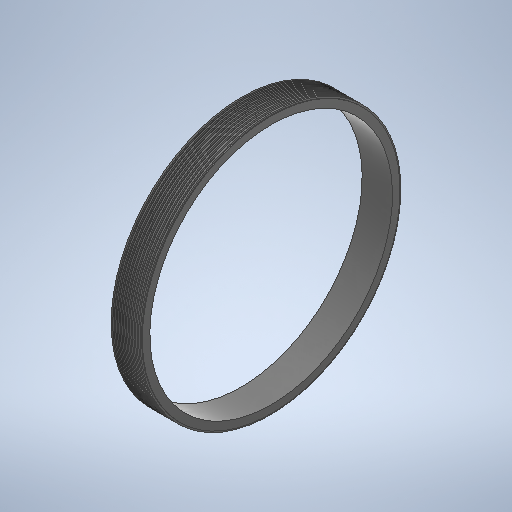
# Autodesk Inventor part: TPU Tire
Saved by Autodesk Inventor 2025.2 (Build 292293000, 293)
## iProperties
Created: 2025-01-18
Part Number: TPU Tire
Material: Generic
Document SubType Name: Modeling
Designer: mtidd
Density: 1 g/cm^3
Appearance: Default
Author: mtidd
Autodesk Inventor part; units mm, degrees
ref_plane "YZ Plane" through (0, 0, 0) normal (1, 0, 0) x (0, 1, 0)
ref_plane "XZ Plane" through (0, 0, 0) normal (0, 1, 0) x (-1, 0, 0)
ref_plane "XY Plane" through (0, 0, 0) normal (0, 0, 1) x (1, 0, 0)
sketch "Sketch1" plane through (0, 0, 0) normal (0, 0, 1) x (1, 0, 0)
  line L0 (-10, 0) -> (-10, 5)
  line L1 (-10, 5) -> (10, 5)
  line L2 (10, 5) -> (10, 0)
  line L3 (10, 0) -> (-10, 0)
  line L4 (-9.5, 5) -> (-8.5, 5)
  line L5 (-8.5, 5) -> (-8.5, 6)
  line L6 (-8.5, 6) -> (-9.5, 6)
  line L7 (-9.5, 6) -> (-9.5, 5)
  line L8 (-6.5, 5) -> (-6.5, 6)
  line L9 (-7.5, 6) -> (-7.5, 5)
  line L10 (-6.5, 6) -> (-7.5, 6)
  line L11 (-4.5, 5) -> (-4.5, 6)
  line L12 (-5.5, 6) -> (-5.5, 5)
  line L13 (-4.5, 6) -> (-5.5, 6)
  line L14 (-2.5, 5) -> (-2.5, 6)
  line L15 (-3.5, 6) -> (-3.5, 5)
  line L16 (-2.5, 6) -> (-3.5, 6)
  line L17 (-0.5, 5) -> (-0.5, 6)
  line L18 (-1.5, 6) -> (-1.5, 5)
  line L19 (-0.5, 6) -> (-1.5, 6)
  line L20 (1.5, 5) -> (1.5, 6)
  line L21 (0.5, 6) -> (0.5, 5)
  line L22 (1.5, 6) -> (0.5, 6)
  line L23 (3.5, 5) -> (3.5, 6)
  line L24 (2.5, 6) -> (2.5, 5)
  line L25 (3.5, 6) -> (2.5, 6)
  line L26 (5.5, 5) -> (5.5, 6)
  line L27 (4.5, 6) -> (4.5, 5)
  line L28 (5.5, 6) -> (4.5, 6)
  line L29 (7.5, 5) -> (7.5, 6)
  line L30 (6.5, 6) -> (6.5, 5)
  line L31 (7.5, 6) -> (6.5, 6)
  line L32 (9.5, 5) -> (9.5, 6)
  line L33 (8.5, 6) -> (8.5, 5)
  line L34 (9.5, 6) -> (8.5, 6)
  point P0 (0, 0)
  point P1 (0, -80)
  dimension "d0" = 5
  dimension "d1" = 20
  dimension "d2" = 90
  dimension "d10" = 1
  dimension "d11" = 1
  dimension "d14" = 2
  constraints: 68 end point, 36 horizontal alignment, 20 parallel, 9 collinear, 3 vertical, 2 perpendicular, 1 horizontal, 4 other
  measures "d0" distance of L0.start L0.end
  measures "d1" distance of L0.end L2.start
  measures "d2" angle to the sketch x axis of L0
  measures "d10" distance of L6.end L5.end
  measures "d11" distance of L5.end L4.end
  measures "d14" distance of L4.end L8.start
sketch "Sketch2" plane through (0, 0, 0) normal (0, 0, 1) x (1, 0, 0)
  line L0 (0, -80.0206) -> (52.1093, -80.0206) construction
  point P0 (0, 0)
  constraints: 2 end point, 1 horizontal
revolve "Revolution1" add sketch "Sketch1" angle 360 about axis through (0, -80.0206, 0) along (1, 0, 0)
body "Solid1"
